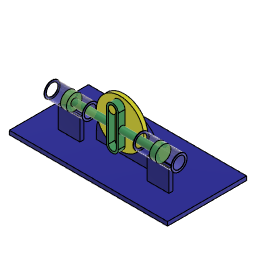
Scotch Yoke Mechanism (Autodesk Fusion 360 design; units mm, degrees)
Autodesk Fusion 360 part; units mm, degrees
note: some values were not read from the file. Set by a fixed rule: which sketch regions a step uses.
ref_plane "WorkPlane1" through (0, 0, 15) normal (0, 0, 1) x (1, 0, 0) in component "Holder"
sketch "Holder base" plane through (0, 0, 15) normal (0, 0, 1) x (1, 0, 0) in component "Holder"
  line L0 (200, 100) -> (-200, 100)
  line L1 (-200, 100) -> (-200, -100)
  line L2 (-200, -100) -> (200, -100)
  line L3 (200, -100) -> (200, 100)
  line L4 (200, 100) -> (-200, -100) construction
  line L5 (-200, 100) -> (200, -100) construction
  line L6 (-200, -100) -> (-170, -100) construction
  line L7 (-200, -100) -> (-200, -70) construction
  line L8 (-200, -70) -> (-170, -70) construction
  circle A0 centre (-170, -70) radius 15
  line L9 (0, 100) -> (0, -100) construction
  line L10 (-200, 0) -> (200, 0) construction
  circle A1 centre (-170, 70) radius 15
  circle A2 centre (170, -70) radius 15
  circle A3 centre (170, 70) radius 15
  line L11 (-200, 0) -> (-70, 0) construction
  line L12 (200, 0) -> (70, 0) construction
  line L13 (70, 10) -> (-70, 10)
  line L14 (-70, 10) -> (-70, -10)
  line L15 (-70, -10) -> (70, -10)
  line L16 (70, -10) -> (70, 10)
  line L17 (70, 10) -> (-70, -10) construction
  line L18 (-70, 10) -> (70, -10) construction
  line L19 (-200, 0) -> (-190, 0) construction
  line L20 (200, 0) -> (190, 0) construction
  dimension "d2" = 400
  dimension "d3" = 200
  dimension "d4" = 30
  dimension "d5" = 30
  dimension "d6" = 30
  dimension "d7" = 130
  dimension "d8" = 130
  dimension "d26" = 10
  dimension "d27" = 10
  constraint horizontal L0
  constraint perpendicular L0 L1
  constraint parallel L0 L2
  constraint parallel L1 L3
  constraint coincident L4 origin
  constraint coincident L5 origin
  constraint perpendicular L1 L6
  constraint perpendicular L2 L7
  constraint perpendicular L7 L8
  constraint coincident L8.end A0.centre
  constraint midpoint L0 L9.start
  constraint midpoint L2 L9.end
  constraint midpoint L1 L10.start
  constraint midpoint L3 L10.end
  constraint symmetric A0 L10 A1
  constraint symmetric A0 L9 A2
  constraint symmetric L9 A1 A3
  constraint perpendicular L1 L11
  constraint perpendicular L3 L12
  constraint horizontal L13
  constraint perpendicular L13 L14
  constraint parallel L13 L15
  constraint parallel L14 L16
  constraint coincident L17 origin
  constraint coincident L18 origin
  constraint perpendicular L1 L19
  constraint coincident L12 L20.end
  measures "d2" distance of L1.end L2.end
  measures "d3" distance of L0.end L1.end
  measures "d4" distance of L1.end L6.end
  measures "d5" distance of L1.end L7.end
  measures "d6" diameter of A0
  measures "d7" distance of L10.start L11.end
  measures "d8" distance of L10.end L12.end
  measures "d26" distance of L10.start L19.end
  measures "d27" distance of L10.end L20.end
extrude "Extrude1" add sketch "Holder base" along normal blind 10 contours L0 L1 L2 L3 | A0 | A1 | A2 | A3 | L13 L14 L15 L16 makes body 1 in component "Holder"
extrude "Extrude2" add sketch "Holder base" against normal blind 15 contours A0 | A1 | A2 | A3 bodies 1 in component "Holder"
extrude "Extrude3" add sketch "Holder base" along normal blind 100 contours L13 L14 L15 L16 bodies 1 in component "Holder"
sketch "Crank" plane through (0, -10, 0) normal (0, -1, 0) x (1, 0, 0) in component "Crank"
  line L0 (-70, 25) -> (70, 25)
  line L1 (70, 25) -> (70, 115)
  line L2 (70, 115) -> (-70, 115)
  line L3 (-70, 115) -> (-70, 25)
  circle A0 centre (0, 100) radius 60
  dimension "d15" = 120
  measures "d15" diameter of A0
extrude "Extrude1'" add sketch "Crank" along normal blind 10 separate body contours L2 A0 | L2 A0 makes body 2 in component "Crank"
sketch "Holder" plane through (0, -20, 0) normal (0, -1, 0) x (1, 0, 0) in component "Crank"
  circle A0 centre (0, 100) radius 60
  circle A1 centre (0, 100) radius 7.5
  dimension "d18" = 15
  constraint concentric A0 A1
  measures "d18" diameter of A1
extrude "Extrude2'" cut sketch "Holder" against normal blind 50 contours A1 bodies 2 in component "Crank"
extrude "Extrude4" add sketch "Holder" along normal blind -10 and the other way blind -2 contours A1 bodies 1 in component "Holder"
move_face "OffsetFaces1" offset -0.3 1 faces at (7.4627, -18, 99.2532) on bodies 1 in component "Holder"
ref_plane "WorkPlane1" through (0, -25, 100) normal (0, -1, 0) x (1, 0, 0) in component "Slider"
sketch "Slider" plane through (0, -25, 100) normal (0, -1, 0) x (1, 0, 0) in component "Slider"
  line L0 (10, 50) -> (-10, 50)
  line L1 (-10, 50) -> (-10, -50)
  line L2 (-10, -50) -> (10, -50)
  line L3 (10, -50) -> (10, 50)
  line L4 (10, 50) -> (-10, -50) construction
  line L5 (-10, 50) -> (10, -50) construction
  line L6 (15, 55) -> (-15, 55)
  line L7 (-15, 55) -> (-15, -55)
  line L8 (-15, -55) -> (15, -55)
  line L9 (15, -55) -> (15, 55)
  line L10 (15, 55) -> (-15, -55) construction
  line L11 (-15, 55) -> (15, -55) construction
  circle A0 centre (0, -40) radius 10
  circle A1 centre (0, -40) radius 15
  circle A2 centre (0, 40) radius 10
  circle A3 centre (0, 40) radius 15
  constraint horizontal L0
  constraint perpendicular L0 L1
  constraint parallel L0 L2
  constraint parallel L1 L3
  constraint coincident L4 origin
  constraint coincident L5 origin
  constraint horizontal L6
  constraint perpendicular L6 L7
  constraint parallel L6 L8
  constraint parallel L7 L9
  constraint coincident L10 origin
  constraint coincident L11 origin
  constraint tangent L3 A0
  constraint concentric A0 A1
  constraint tangent L9 A1
  constraint tangent L3 A2
  constraint concentric A2 A3
  constraint tangent L9 A3
extrude "Extrude1''" add sketch "Slider" along normal blind 15 and the other way blind 2 separate body contours L0 L3 A2 | L0 L1 L3 A3 | L0 L1 A2 | L3 L9 A1 A3 | L1 L7 A1 A3 | L1 L2 L3 A1 | L2 L3 A0 | L1 L2 A0 makes body 3 in component "Slider"
fillet "Fillet1" radius 70 1 edges at (70, 0, 115) on bodies 1 in component "Holder"
fillet "Fillet2" radius 70 1 edges at (-70, 0, 115) on bodies 1 in component "Holder"
sketch "Right side" plane through (15, 0, 0) normal (1, 0, 0) x (0, 1, 0) in component "Slider"
  line L0 (-23, 140) -> (-40, 140)
  line L1 (-40, 140) -> (-40, 60)
  line L2 (-40, 60) -> (-23, 60)
  line L3 (-23, 60) -> (-23, 140)
  circle A0 centre (-31.5, 100) radius 8.5
  constraint tangent L1 A0
extrude "Extrude2''" add sketch "Right side" along normal blind 90 contours A0 bodies 3 in component "Slider"
sketch "Right piston" plane through (105, 0, 0) normal (1, 0, 0) x (0, 1, 0) in component "Slider"
  circle A0 centre (-31.5, 100) radius 8.5
  circle A1 centre (-31.5, 100) radius 20
  dimension "d37" = 40
  constraint concentric A0 A1
  measures "d37" diameter of A1
extrude "Extrude6" add sketch "Right piston" along normal blind 15 contours A0 | A1 bodies 3 in component "Slider"
ref_plane "WorkPlane2" through (75, -31.5, 100) normal (1, 0, 0) x (0, 1, 0) in component "Holder"
sketch "Right piston holder left" plane through (75, -31.5, 100) normal (1, 0, 0) x (0, 1, 0) in component "Holder"
  circle A0 centre (0, 0) radius 20.15
  circle A1 centre (0, 0) radius 20.15
  circle A2 centre (0, 0) radius 16.1245
  line L0 (0, 0) -> (0, 20.15) construction
  line L1 (0, 0) -> (0, -20.15) construction
  dimension "d41" = 40.3
  constraint coincident A0.centre A1.centre
  constraint concentric A0 A1
  constraint concentric A1 A2
  constraint coincident A0 L0.end
  constraint vertical L0
  constraint coincident A0 L1.end
  constraint parallel L0 L1
  measures "d41" diameter of A0
extrude "Extrude5" add sketch "Right piston holder left" along normal blind 75 separate body contours A0 A1 | A2 makes body 4 in component "Holder"
hole "Hole1" at (150, -31.5, 100) direction (-1, 0, 0) diameter 40 depth 95 tip angle 180 bodies 4 in component "Holder"
ref_plane "WorkPlane3" through (150, -31.5, 100) normal (1, 0, 0) x (0, 1, 0) in component "Holder"
sketch "Right piston holder right" plane through (150, -31.5, 100) normal (1, 0, 0) x (0, 1, 0) in component "Holder"
  circle A0 centre (0, 0) radius 16.1245
  circle A1 centre (0, 0) radius 19.8494
  line L0 (0, 0) -> (0, 19.8494) construction
  line L1 (0, 0) -> (0, -19.8494) construction
  line L2 (0, -19.8494) -> (0, -75) construction
  circle A2 centre (0, 0) radius 20.1619
  constraint coincident A0.centre A1.centre
  constraint coincident A1 L0.end
  constraint vertical L0
  constraint coincident A1 L1.end
  constraint parallel L0 L1
  constraint parallel L1 L2
ref_plane "WorkPlane4" through (150, -31.5, 100) normal (0, -1, 0) x (1, 0, 0) in component "Holder"
sketch "Right holder piston" plane through (150, -31.5, 100) normal (0, -1, 0) x (1, 0, 0) in component "Holder"
  line L0 (-65, -20) -> (-10, -20)
  line L1 (-10, -20) -> (-10, -75)
  line L2 (-10, -75) -> (-65, -75)
  line L3 (-65, -75) -> (-65, -20)
  constraint horizontal L0
  constraint vertical L1
  constraint horizontal L2
  constraint vertical L3
extrude "Extrude9" add sketch "Right holder piston" along normal mid plane 10 bodies 4 1 in component "Holder"
sketch "Left side" plane through (-15, 0, 0) normal (-1, 0, 0) x (0, -1, 0) in component "Slider"
  line L0 (23, 60) -> (40, 60)
  line L1 (40, 60) -> (40, 140)
  line L2 (40, 140) -> (23, 140)
  line L3 (23, 140) -> (23, 60)
  circle A0 centre (31.5012, 100) radius 8.4988
  constraint tangent L1 A0
extrude "Extrude4'" add sketch "Left side" along normal blind 90 contours A0 bodies 3 in component "Slider"
sketch "Left piston" plane through (-105, 0, 0) normal (-1, 0, 0) x (0, -1, 0) in component "Slider"
  circle A0 centre (31.5012, 100) radius 8.4988
  circle A1 centre (31.5012, 100) radius 20
  dimension "d61" = 40
  constraint concentric A0 A1
  measures "d61" diameter of A1
extrude "Extrude5'" add sketch "Left piston" along normal blind 15 contours A0 | A1 bodies 3 in component "Slider"
move_face "OffsetFaces2" offset -0.3 1 faces at (-115, -51.4018, 98.0086) on bodies 3 in component "Slider"
move_face "OffsetFaces4" offset -0.3 1 faces at (115, -11.5994, 98.0086) on bodies 3 in component "Slider"
ref_plane "WorkPlane5" through (-75, -31.5012, 100) normal (-1, 0, 0) x (0, -1, 0) in component "Holder"
sketch "Left holder piston right" plane through (-75, -31.5012, 100) normal (-1, 0, 0) x (0, 1, 0) in component "Holder"
  circle A0 centre (0, 0) radius 20
  circle A1 centre (0, 0) radius 16.1245
  line L0 (0, 0) -> (0, -20) construction
  dimension "d70" = 40
  constraint coincident A0.centre A1.centre
  constraint concentric A0 A1
  constraint coincident A0 L0.end
  constraint vertical L0
  measures "d70" diameter of A0
extrude "Extrude11" add sketch "Left holder piston right" along normal blind 75 separate body contours A0 | A1 makes body 5 in component "Holder"
hole "Hole2" at (-150, -31.5012, 100) direction (1, 0, 0) diameter 39.7 depth 79 tip angle 180 bodies 5 in component "Holder"
ref_plane "WorkPlane6" through (-150, -31.5012, 100) normal (-1, 0, 0) x (0, -1, 0) in component "Holder"
sketch "Left holder piston left" plane through (-150, -31.5012, 100) normal (-1, 0, 0) x (0, 1, 0) in component "Holder"
  circle A0 centre (0, 0) radius 16.0456
  circle A1 centre (0, 0) radius 20
  line L0 (0, 0) -> (0, -20) construction
  line L1 (0, 20) -> (0, 75) construction
  constraint coincident A0.centre A1.centre
  constraint coincident A1 L0.end
  constraint vertical L0
  constraint coincident A1 L1.start
  constraint parallel L0 L1
ref_plane "WorkPlane7" through (-150, -31.5012, 100) normal (0, -1, 0) x (1, 0, 0) in component "Holder"
sketch "Left holder piston" plane through (-150, -31.5012, 100) normal (0, -1, 0) x (1, 0, 0) in component "Holder"
  line L0 (0, -75) -> (10, -75) construction
  line L1 (10, -75) -> (65, -75)
  line L2 (65, -75) -> (65, -20)
  line L3 (65, -20) -> (10, -20)
  line L4 (10, -20) -> (10, -75)
  dimension "d81" = 10
  constraint horizontal L0
  constraint horizontal L1
  constraint vertical L2
  constraint horizontal L3
  constraint vertical L4
  measures "d81" distance of L0.start L0.end
extrude "Extrude14" add sketch "Left holder piston" along normal mid plane 10 bodies 4 5 in component "Holder"
sketch "Contact point" plane through (0, -20, 0) normal (0, -1, 0) x (1, 0, 0) in component "Crank"
  circle A0 centre (0, 100) radius 7.5
  circle A1 centre (0, 100) radius 60
  circle A2 centre (0, 140) radius 9.5
  dimension "d84" = 19
  measures "d84" diameter of A2
extrude "Extrude3'" add sketch "Contact point" along normal blind 20 contours A2 bodies 2 in component "Crank"
extrude "Extrude15" add 1 faces at (-150, -21.5697, 82.7981) along direction (-1, 0, 0) blind 10 on bodies 4 bodies 4 in component "Holder"
extrude "Extrude16" add 1 faces at (-75, -21.5697, 82.7981) along direction (1, 0, 0) blind 10 on bodies 4 bodies 4 in component "Holder"
extrude "Extrude17" add 1 faces at (75, -24.1885, 118.6293) along direction (-1, 0, 0) blind 10 on bodies 4 bodies 4 in component "Holder"
extrude "Extrude18" add 1 faces at (150, -24.1885, 118.6293) along direction (1, 0, 0) blind 10 on bodies 4 bodies 4 in component "Holder"
ref_plane "WorkPlane8" through (160, -31.5, 100) normal (1, 0, 0) x (0, 1, 0) in component "Holder"
sketch "Right piston holder right (1)" plane through (160, -31.5, 100) normal (1, 0, 0) x (0, 1, 0) in component "Holder"
  circle A0 centre (0, 0) radius 15
  circle A1 centre (0, 0) radius 20
  dimension "d104" = 30
  dimension "d105" = 40
  constraint coincident A0.centre A1.centre
  constraint concentric A0 A1
  measures "d104" diameter of A0
  measures "d105" diameter of A1
extrude "Extrude19" add sketch "Right piston holder right (1)" along normal blind 1 bodies 4 in component "Holder"
ref_plane "WorkPlane9" through (65, -31.5, 100) normal (-1, 0, 0) x (0, -1, 0) in component "Holder"
sketch "Right piston holder left (1)" plane through (65, -31.5, 100) normal (-1, 0, 0) x (0, 1, 0) in component "Holder"
  circle A0 centre (0, 0) radius 15
  circle A1 centre (0, 0) radius 20
  dimension "d109" = 30
  dimension "d110" = 40
  constraint coincident A0.centre A1.centre
  constraint concentric A0 A1
  measures "d109" diameter of A0
  measures "d110" diameter of A1
extrude "Extrude20" add sketch "Right piston holder left (1)" along normal blind 1 bodies 4 in component "Holder"
ref_plane "WorkPlane10" through (-160, -31.5012, 100) normal (-1, 0, 0) x (0, -1, 0) in component "Holder"
sketch "Left holder piston left (1)" plane through (-160, -31.5012, 100) normal (-1, 0, 0) x (0, 1, 0) in component "Holder"
  circle A0 centre (0, 0) radius 15
  circle A1 centre (0, 0) radius 20
  dimension "d114" = 30
  dimension "d115" = 40
  constraint coincident A0.centre A1.centre
  measures "d114" diameter of A0
  measures "d115" diameter of A1
extrude "Extrude21" add sketch "Left holder piston left (1)" along normal blind 1 bodies 4 in component "Holder"
ref_plane "WorkPlane11" through (-65, -31.5012, 100) normal (1, 0, 0) x (0, 1, 0) in component "Holder"
sketch "Left holder piston right (1)" plane through (-65, -31.5012, 100) normal (1, 0, 0) x (0, 1, 0) in component "Holder"
  circle A0 centre (0, 0) radius 15
  circle A1 centre (0, 0) radius 20
  dimension "d119" = 30
  dimension "d120" = 40
  constraint coincident A0.centre A1.centre
  constraint concentric A0 A1
  measures "d119" diameter of A0
  measures "d120" diameter of A1
extrude "Extrude22" add sketch "Left holder piston right (1)" along normal blind 1 bodies 4 in component "Holder"
component "Holder" placed x (1, 0, 0) y (0, 1, 0) z (0, 0, 1) at (0, 0, 0)
component "Crank" placed x (1, 0, 0) y (0, 1, 0) z (0, 0, 1) at (0, 0, 0)
component "Slider" placed x (1, 0, 0) y (0, 1, 0) z (0, 0, 1) at (0, 0, 0)
equation "d74 = 40.00 mm - 0.3 mm"
named bodies: "Holder", "Crank", "Slider"
